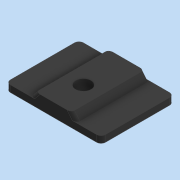
# Autodesk Inventor part: 0 零件
Saved by Autodesk Inventor 2020 (Build 240168000, 168)
## iProperties
Created: 2020-11-03
Part Number: 0 零件
Material: 橡膠
Document SubType Name: Modeling
Designer: p2013
Density: 0.93 g/cm^3
Appearance: 橡膠 - 黑色
Author: p2013
Autodesk Inventor part; units mm, degrees
ref_plane "YZ Plane" through (0, 0, 0) normal (1, 0, 0) x (0, 1, 0)
ref_plane "XZ Plane" through (0, 0, 0) normal (0, 1, 0) x (-1, 0, 0)
ref_plane "XY Plane" through (0, 0, 0) normal (0, 0, 1) x (1, 0, 0)
sketch "草圖1" plane through (0, 0, 0) normal (0, 0, 1) x (1, 0, 0)
  line L0 (0, 0) -> (-21.5, 0) construction
  line L1 (0, 0) -> (0, 14.995) construction
  line L2 (-21.5, 0) -> (-21.5, 3)
  line L3 (-21.5, 3) -> (-10.5, 3)
  line L4 (-10.5, 3) -> (-8, 6)
  line L5 (21.5, 0) -> (21.5, 3)
  line L6 (21.5, 3) -> (10.5, 3)
  line L7 (10.5, 3) -> (8, 6)
  line L8 (-8, 6) -> (8, 6)
  line L9 (-21.5, 0) -> (21.5, 0)
  dimension "d0" = 3
  dimension "d1" = 16
  dimension "d2" = 43
  dimension "d3" = 11
  dimension "d4" = 6
  constraints: 20 end point, 4 symmetric about line, 2 horizontal, 2 perpendicular, 2 vertical
  measures "d0" distance between parallel lines of L6 L9
  measures "d1" distance of L4.end L7.end
  measures "d2" distance between parallel lines of L2 L5
  measures "d3" distance of L5.end L6.end
  measures "d4" distance between parallel lines of L9 L8
extrude "擠出1" add sketch "草圖1" along normal mid plane 33
fillet "圓角1" radius 1.5 4 edges at (9.25, 4.5, 16.5) (9.25, 4.5, -16.5) (-9.25, 4.5, 16.5) (-9.25, 4.5, -16.5)
fillet "圓角2" radius 2 4 edges at (21.5, 1.5, 16.5) (21.5, 1.5, -16.5) (-21.5, 1.5, -16.5) (-21.5, 1.5, 16.5)
sketch "草圖3" plane through (-19.5, 0, -16.5) normal (0, -1, 0) x (1, 0, 0)
  line L0 (0, 33) -> (39, 33) projected
  line L1 (19.5, 19.5) -> (19.5, 33) construction
  circle A0 centre (18, 30) radius 0.75
  point P0 (19.5, 16.5)
  dimension "d13" = 1.5
  dimension "d14" = 3
  dimension "d15" = 1.5
  constraints: 2 end point, 1 centre point, 1 midpoint
  measures "d13" diameter of A0
  measures "d14" distance from line of A0.centre L0
  measures "d15" distance from line of A0.centre L1
extrude "擠出3" add sketch "草圖3" along normal blind 1
pattern_linear "矩形陣列1" count 7 spacing 3 along (-1, 0, 0) count 10 spacing 3 along (0, 0, -1) of "擠出3"
mirror "鏡射1" about plane through (0, 0, 0) normal (1, 0, 0) of "擠出3", "矩形陣列1"
sketch "草圖4" plane through (-6.0474, 6, 16.5) normal (0, 1, 0) x (1, 0, 0)
  line L0 (12.0949, 0) -> (0, 0) projected
  circle A0 centre (6.0474, 13.5) radius 3.5
  point P0 (6.0474, 16.5)
  dimension "d24" = 7
  dimension "d25" = 13.5
  constraints: 1 centre point, 1 vertical alignment
  measures "d24" diameter of A0
  measures "d25" distance from line of L0 A0.centre
extrude "擠出4" cut sketch "草圖4" against normal through all
